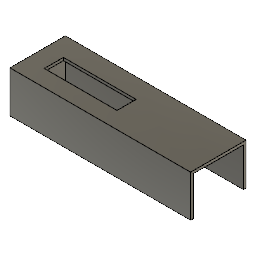
controls v1 (Autodesk Fusion 360 design; units mm, degrees)
Autodesk Fusion 360 part; units mm, degrees
note: some values were not read from the file. Set by a fixed rule: which face or edge a step refers to.
sketch "Sketch1" plane through (0, 0, 0) normal (0, 0, 1) x (1, 0, 0)
  line L0 (-25, 10) -> (25, 10)
  line L1 (25, 10) -> (25, -10)
  line L2 (25, -10) -> (-25, -10)
  line L3 (-25, -10) -> (-25, 10)
  dimension "d1" = 50
  constraint horizontal L0
  constraint vertical L1
  constraint horizontal L2
  constraint vertical L3
  measures "d1" distance of L0.start L0.end
extrude "Extrude1" add sketch "Sketch1" along normal blind 15
shell "Shell1" thickness 1 removed faces 1 at (-8.3333, 3.3333, 0)
ref_plane "WorkPlane1" through (0, 0, 30) normal (0, 0, 1) x (1, 0, 0)
sketch "Sketch2" plane through (0, 0, 30) normal (0, 0, 1) x (1, 0, 0)
  line L0 (-18.5665, 2.8665) -> (7.5566, 2.8665)
  line L1 (7.5566, 2.8665) -> (7.5566, -4.0069)
  line L2 (7.5566, -4.0069) -> (-18.5665, -4.0069)
  line L3 (-18.5665, -4.0069) -> (-18.5665, 2.8665)
  constraint horizontal L0
  constraint vertical L1
  constraint horizontal L2
  constraint vertical L3
extrude "Extrude2" cut sketch "Sketch2" against normal blind 45
move_face "OffsetFaces2" offset 15 1 faces at (25, 3.3333, 5)
delete_face "DeleteFace1" 1 faces at (24, 3, 9.3333)
move_face "OffsetFaces1" [rolled back] distance 15
